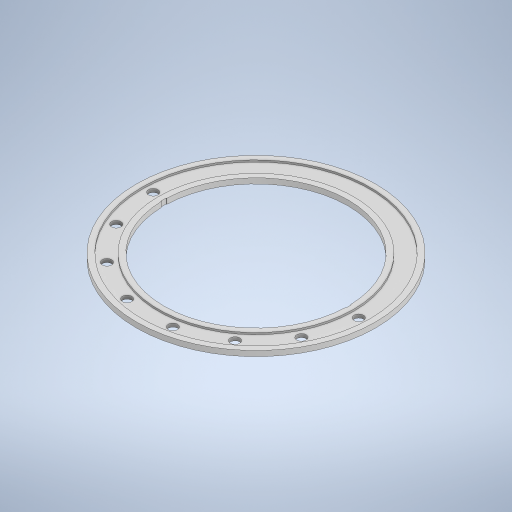
# Autodesk Inventor part: ДМС 020 кольцо прижимное 1
Saved by Autodesk Inventor 2024.2 (Build 282272000, 272)
## iProperties
Created: 2024-04-23
Part Number: ДМС 020 кольцо прижимное 1
Material: Generic
Document SubType Name: Modeling
Designer: admin
Density: 1 g/cm^3
Appearance: Default
Author: admin
Autodesk Inventor part; units mm, degrees
ref_plane "YZ Plane" through (0, 0, 0) normal (1, 0, 0) x (0, 1, 0)
ref_plane "XZ Plane" through (0, 0, 0) normal (0, 1, 0) x (-1, 0, 0)
ref_plane "XY Plane" through (0, 0, 0) normal (0, 0, 1) x (1, 0, 0)
sketch "Sketch1" plane through (0, 0, 0) normal (0, 0, 1) x (1, 0, 0)
  circle A0 centre (0, 0) radius 174
  circle A1 centre (0, 0) radius 226
  circle A2 centre (0, 0) radius 200 construction
  line L0 (0, 174) -> (0, 226) construction
  point P0 (0, 200)
  dimension "d17" = 400
  dimension "d18" = 52
  constraints: 4 vertical alignment, 3 coincident, 2 end point, 1 midpoint, 1 vertical, 6 other
  measures "d18" distance of L0.start L0.end
extrude "Extrusion1" add sketch "Sketch1" along normal blind 10
sketch "Sketch2" plane through (0, 0, 10) normal (0, 0, 1) x (1, 0, 0)
  circle A0 centre (0, 0) radius 226 construction
  circle A1 centre (0, 0) radius 174 construction
  line L0 (0, 215.5) -> (0, 184.5) construction
  line L1 (0, 174) -> (0, 0) construction
  circle A2 centre (0, 0) radius 184.5
  circle A3 centre (0, 0) radius 215.5
  circle A4 centre (0, 0) radius 200 construction
  point P0 (0, 200)
  dimension "d19" = 400
  dimension "d4" = 31
  constraints: 5 vertical alignment, 4 end point, 3 coincident, 2 vertical, 1 midpoint, 7 other
  measures "d4" distance of L0.start L0.end
extrude "Extrusion2" cut sketch "Sketch2" against normal blind 3.5
sketch "Sketch3" plane through (0, 0, 0) normal (0, 0, 1) x (1, 0, 0)
  circle A0 centre (0, 0) radius 174 construction
  circle A1 centre (0, 0) radius 226 construction
  circle A2 centre (0, 0) radius 184.5 projected
  circle A3 centre (0, 0) radius 215.5 projected
  circle A4 centre (0, 0) radius 226 projected
  line L0 (0, 0) -> (0, -226) construction
  line L1 (0, 0) -> (44.0904, -221.6575) construction
  line L2 (35.9942, -180.9549) -> (42.042, -211.3592) construction
  circle A5 centre (39.0181, -196.1571) radius 9
  dimension "d20" = 11.25
  dimension "d21" = 18
  constraints: 6 end point, 2 point on circle, 2 point on line, 1 centre point, 1 midpoint, 1 vertical, 4 other
  measures "d20" angle of L1 L0
  measures "d21" diameter of A5
extrude "Extrusion3" cut sketch "Sketch3" along normal through all contours A5
pattern_circular "Circular Pattern2" count 8 over 180 about axis through (0, 0, 0) along (0, 0, -1) of "Extrusion3" both ways yes
sketch "Sketch5" plane through (0, 0, 0) normal (0, 0, -1) x (-1, 0, 0)
  circle A0 centre (0, 0) radius 174 projected
  circle A1 centre (0, 0) radius 226 projected
  line L0 (174, 0) -> (175, 0) construction
  line L1 (175, 5) -> (175, -5)
  line L2 (175, 5) -> (173.9281, 5)
  line L3 (175, -5) -> (173.9281, -5)
  line L4 (-174, 0) -> (-175, 0) construction
  line L5 (-175, 5) -> (-175, -5)
  line L6 (-175, 5) -> (-173.9281, 5)
  line L7 (-175, -5) -> (-173.9281, -5)
  dimension "d32" = 10
  dimension "d33" = 1
  constraints: 16 end point, 6 horizontal, 6 point on circle, 2 equal length, 2 horizontal alignment, 2 midpoint, 2 vertical
  measures "d32" distance of L1.start L1.end
  measures "d33" distance of L0.start L0.end
extrude "Extrusion4" cut sketch "Sketch5" against normal through all contours A0 L2 L1 L3 | A0 L7 L5 L6
equation "\"d17\" = Шпил_пласт_НОС_диам_центров"
equation "\"d19\" = Шпил_пласт_НОС_диам_центров"
equation "\"Шпил_пласт_НОС_диам_центров\" = 400"
body "Solid1"
